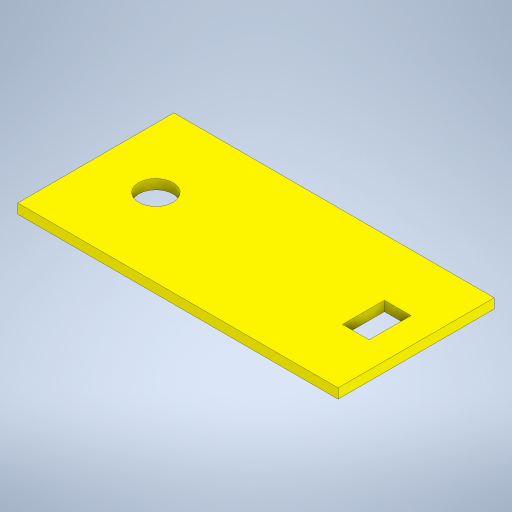
# Autodesk Inventor part: PARED
Saved by Autodesk Inventor 2024 (Build 280153000, 153)
## iProperties
Created: 2024-05-05
Part Number: PARED
Material: Generic
Document SubType Name: Modeling
Designer: samue
Density: 1 g/cm^3
Appearance: Default
Author: samue
Autodesk Inventor part; units mm, degrees
ref_plane "YZ Plane" through (0, 0, 0) normal (1, 0, 0) x (0, 1, 0)
ref_plane "XZ Plane" through (0, 0, 0) normal (0, 1, 0) x (-1, 0, 0)
ref_plane "XY Plane" through (0, 0, 0) normal (0, 0, 1) x (1, 0, 0)
sketch "Sketch1" plane through (0, 0, 0) normal (0, 1, 0) x (-1, 0, 0)
  line L0 (51.3, 25) -> (-51.3, 25)
  line L1 (-51.3, 25) -> (-51.3, -25)
  line L2 (-51.3, -25) -> (51.3, -25)
  line L3 (51.3, -25) -> (51.3, 25)
  line L4 (51.3, 25) -> (-51.3, -25) construction
  line L5 (-51.3, 25) -> (51.3, -25) construction
  point P0 (0, 0)
  dimension "d0" = 102.6
  dimension "d1" = 50
  constraints: 12 end point, 2 midpoint, 2 parallel, 1 horizontal, 1 perpendicular
  measures "d0" distance of L2.end L1.end
  measures "d1" distance of L1.end L0.end
extrude "Extrusion1" add sketch "Sketch1" along normal blind 3.125
sketch "Sketch2" plane through (0, 3.125, 0) normal (0, 1, 0) x (1, 0, 0)
  circle A0 centre (-32.0787, 0) radius 5.5
  point P0 (0, 0)
  dimension "d4" = 11
  constraints: 1 centre point
  measures "d4" diameter of A0
extrude "Extrusion2" cut sketch "Sketch2" against normal blind 3.125
sketch "Sketch3" plane through (0, 3.125, 0) normal (0, 1, 0) x (1, 0, 0)
  line L0 (34.4414, -6.7) -> (42.9414, -6.7)
  line L1 (42.9414, -6.7) -> (42.9414, 6.7)
  line L2 (42.9414, 6.7) -> (34.4414, 6.7)
  line L3 (34.4414, 6.7) -> (34.4414, -6.7)
  line L4 (34.4414, -6.7) -> (42.9414, 6.7) construction
  line L5 (42.9414, -6.7) -> (34.4414, 6.7) construction
  point P0 (0, 0)
  point P1 (38.6914, 0)
  dimension "d7" = 8.5
  dimension "d8" = 13.4
  constraints: 12 end point, 2 midpoint, 2 parallel, 1 horizontal, 1 perpendicular
  measures "d7" distance of L2.end L1.end
  measures "d8" distance of L1.end L0.end
extrude "Extrusion3" cut sketch "Sketch3" against normal blind 3.125
body "Solid1"
